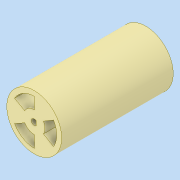
# Autodesk Inventor part: 滚轮内轮
Saved by Autodesk Inventor 2019 (Build 230136000, 136)
## iProperties
Created: 2020-11-02
Part Number: 滚轮内轮
Material: 尼龙 6/6
Document SubType Name: Modeling
Designer: Wang Hua
Density: 1.13 g/cm^3
Appearance: 尼龙 6
Author: Wang Hua
Autodesk Inventor part; units mm, degrees
ref_plane "YZ Plane" through (0, 0, 0) normal (1, 0, 0) x (0, 1, 0)
ref_plane "XZ Plane" through (0, 0, 0) normal (0, 1, 0) x (-1, 0, 0)
sketch "草图1" plane through (0, 0, 0) normal (0, 0, 1) x (1, 0, 0)
  circle A0 centre (0, 0) radius 15.25
  dimension "d0" = 30.5
  constraints: 1 centre point, 1 coincident
  measures "d0" diameter of A0
extrude "拉伸1" add sketch "草图1" along normal blind 62
sketch "草图2" plane through (0, 0, 62) normal (0, 0, 1) x (1, 0, 0)
  arc A0 (5.1473, -3.0831) -> (5.1473, 3.0831) centre (0, 0) ccw
  arc A1 (10.7235, -6.423) -> (10.7235, 6.423) centre (0, 0) ccw
  line L0 (5.1473, 3.0831) -> (10.7235, 6.423)
  line L1 (0, 0) -> (24.4496, 0) construction
  line L2 (5.1473, -3.0831) -> (10.7235, -6.423)
  line L3 (-5.2437, 2.9162) -> (-10.9243, 6.0753)
  arc A2 (0.0964, 5.9992) -> (-5.2437, 2.9162) centre (0, 0) ccw
  line L4 (0.0964, 5.9992) -> (0.2008, 12.4984)
  arc A3 (0.2008, 12.4984) -> (-10.9243, 6.0753) centre (0, 0) ccw
  line L5 (0.0964, -5.9992) -> (0.2008, -12.4984)
  arc A4 (-5.2437, -2.9162) -> (0.0964, -5.9992) centre (0, 0) ccw
  line L6 (-5.2437, -2.9162) -> (-10.9243, -6.0753)
  arc A5 (-10.9243, -6.0753) -> (0.2008, -12.4984) centre (0, 0) ccw
  dimension "d4" = 12
  dimension "d5" = 30.92
  dimension "d8" = 360
  dimension "d16" = 12.5
  constraints: 14 end point, 12 point on circle, 6 centre point, 4 coincident, 2 symmetric about line, 1 horizontal, 31 other
  measures "d4" diameter of A0
  measures "d5" angle of L1 L0
  measures "d16" radius of A1
extrude "拉伸2" cut sketch "草图2" against normal through all
sketch "草图3" plane through (0, 0, 62) normal (0, 0, 1) x (1, 0, 0)
  arc A0 (1, 1.249) -> (1, -1.249) centre (0, 0) ccw
  line L0 (1, 1.249) -> (1, -1.249)
  line L1 (-1.6, 0) -> (-1.6, 2.5625) construction
  dimension "d12" = 3.2
  dimension "d13" = 2.6
  constraints: 4 end point, 3 point on circle, 2 vertical, 1 centre point, 1 coincident
  measures "d12" diameter of A0
  measures "d13" distance from line of L0 L1.start
extrude "拉伸3" cut sketch "草图3" against normal blind 9.2
ref_plane "工作平面1" through (0, 0, 31) normal (0, 0, 1) x (1, 0, 0)
mirror "镜像1" about plane through (0, 0, 31) normal (0, 0, 1) of "拉伸3"
